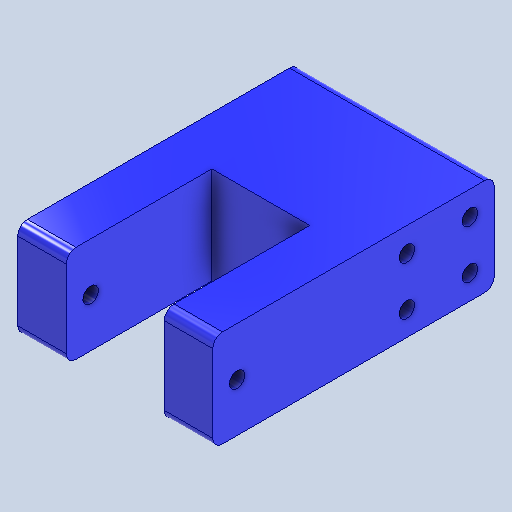
# Autodesk Inventor part: dribl-v1-3DP-cc-f-2
Saved by Autodesk Inventor 2025.2 (Build 292293000, 293)
## iProperties
Created: 2025-03-16
Part Number: dribl-v1-3DP-cc-f-2
Material: ABS プラスチック
Document SubType Name: Modeling
Designer: haruy
Density: 1.06 g/cm^3
Appearance: 青 - 壁塗料 - 光沢
Author: haruy
Autodesk Inventor part; units mm, degrees
ref_plane "YZ Plane" through (0, 0, 0) normal (1, 0, 0) x (0, 1, 0)
ref_plane "XZ Plane" through (0, 0, 0) normal (0, 1, 0) x (-1, 0, 0)
sketch "スケッチ1" plane through (0, 0, 0) normal (1, 0, 0) x (0, 1, 0)
  line L0 (0, 0) -> (37.4755, 0)
  line L1 (37.4755, 0) -> (37.4755, -20)
  line L2 (37.4755, -20) -> (0, -20)
  line L3 (0, -20) -> (0, 0)
  line L4 (9.6981, 10) -> (29.6981, 10)
  line L5 (29.6981, 10) -> (29.6981, -48)
  line L6 (29.6981, -48) -> (9.6981, -48)
  line L7 (9.6981, -48) -> (9.6981, 10)
  circle A0 centre (24.6981, -30) radius 1.6
  circle A1 centre (14.6981, -30) radius 1.6
  circle A2 centre (24.6981, -43) radius 1.6
  circle A3 centre (14.6981, -43) radius 1.6
  circle A4 centre (19.6981, 5) radius 1.6
  point P0 (29.6981, -20)
  point P1 (9.6981, -20)
  dimension "d0" = 20
  dimension "d1" = 10
  dimension "d2" = 3.2
  dimension "d3" = 3.2
  dimension "d4" = 3.2
  dimension "d5" = 3.2
  dimension "d6" = 10
  dimension "d7" = 10
  dimension "d8" = 13
  dimension "d9" = 0
  dimension "d10" = 0
  dimension "d11" = 13
  dimension "d12" = 5
  dimension "d13" = 10
  dimension "d14" = 5
  dimension "d15" = 5
  dimension "d16" = 3.2
  dimension "d17" = 5
  dimension "d18" = 10
  constraints: 16 end point, 5 centre point, 4 parallel, 2 horizontal, 2 perpendicular
  measures "d0" distance of L0.end L1.end
  measures "d1" distance between parallel lines of L4 L0
  measures "d2" diameter of A0
  measures "d3" diameter of A1
  measures "d4" diameter of A2
  measures "d5" diameter of A3
  measures "d6" distance of A1.centre A0.centre
  measures "d7" distance of A3.centre A2.centre
  measures "d8" distance of A2.centre A0.centre
  measures "d9" horizontal distance of A2.centre A0.centre
  measures "d10" vertical distance of A1.centre A0.centre
  measures "d11" distance of A3.centre A1.centre
  measures "d12" distance from line of L6 A2.centre
  measures "d13" distance from line of A0.centre L2
  measures "d14" distance from line of A0.centre L5
  measures "d15" distance from line of L7 A1.centre
  measures "d16" diameter of A4
  measures "d17" distance from line of A4.centre L4
  measures "d18" distance from line of A4.centre L7
extrude "押し出し1" add sketch "スケッチ1" along normal blind 10 contours L7 L4 L5 L0 | L0 L5 L2 L7 | L2 L5 L6 L7
extrude "押し出し2" add sketch "スケッチ1" against normal blind 10.1 contours L2 L5 L6 L7
ref_plane "作業平面1" through (-10.1, 0, 0) normal (-1, 0, 0) x (0, 0, 1)
mirror "ミラー1" about plane through (-10.1, 0, 0) normal (-1, 0, 0)
fillet "フィレット1" radius 2 6 edges at (5, 29.6981, 10) (5, 9.6981, 10) (-25.2, 29.6981, 10) (-25.2, 9.6981, 10) (-10.1, 29.6981, -48) (-10.1, 9.6981, -48)
equation "\"d11\" = d8"
